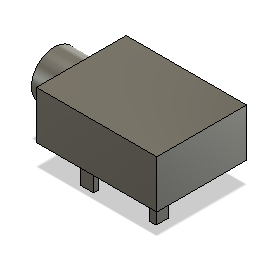
KTANE_game (Autodesk Fusion 360 archive; units mm, degrees)
design "3,5 mm female jack"
Autodesk Fusion 360 part; units mm, degrees
sketch "Sketch1" plane through (0, 0, 0) normal (0, 1, 0) x (1, 0, 0)
  line L0 (7.81, -5.825) -> (-7.81, -5.825)
  line L1 (-7.81, -5.825) -> (-7.81, 5.825)
  line L2 (-7.81, 5.825) -> (7.81, 5.825)
  line L3 (7.81, 5.825) -> (7.81, -5.825)
  line L4 (7.81, -5.825) -> (-7.81, 5.825) construction
  line L5 (-7.81, -5.825) -> (7.81, 5.825) construction
  dimension "d1" = 15.62
  dimension "d2" = 11.65
  constraint horizontal L0
  constraint perpendicular L0 L1
  constraint parallel L0 L2
  constraint parallel L1 L3
  constraint coincident L4 origin
  constraint coincident L5 origin
  measures "d1" distance of L1.end L2.end
  measures "d2" distance of L0.end L1.end
extrude "Extrude1" add sketch "Sketch1" along normal mid plane 6.2
sketch "Sketch2" plane through (-7.81, 0, 0) normal (-1, 0, 0) x (0, 0, 1)
  line L0 (5.825, -3.1) -> (5.825, 3.1)
  line L1 (5.825, 3.1) -> (-5.825, 3.1)
  line L2 (-5.825, 3.1) -> (-5.825, -3.1)
  line L3 (-5.825, -3.1) -> (5.825, -3.1)
  circle A0 centre (0, 0) radius 2.975
  circle A1 centre (0, 0) radius 1.8
  dimension "d5" = 5.95
  dimension "d6" = 3.6
  constraint coincident A0.centre A1.centre
  constraint concentric A0 A1
  measures "d5" diameter of A0
  measures "d6" diameter of A1
extrude "Extrude2" add sketch "Sketch2" along normal blind 3.5 contours A0
sketch "Sketch3" plane through (0, -3.1, 0) normal (0, -1, 0) x (1, 0, 0)
  line L0 (-7.81, -5.825) -> (7.81, -5.825)
  line L1 (7.81, -5.825) -> (7.81, 5.825)
  line L2 (7.81, 5.825) -> (-7.81, 5.825)
  line L3 (-7.81, 5.825) -> (-7.81, -5.825)
  line L4 (-1.1432, 4.3971) -> (-2.81, 4.3971)
  line L5 (-2.81, 4.3971) -> (-2.81, 5.075)
  line L6 (-2.81, 5.075) -> (-1.1432, 5.075)
  line L7 (-1.1432, 5.075) -> (-1.1432, 4.3971)
  line L8 (-1.1432, 4.3971) -> (-2.81, 5.075) construction
  line L9 (-2.81, 4.3971) -> (-1.1432, 5.075) construction
  line L10 (-5.2893, -1.2) -> (-6.2893, -1.2)
  line L11 (-6.2893, -1.2) -> (-6.2893, 1.2)
  line L12 (-6.2893, 1.2) -> (-5.2893, 1.2)
  line L13 (-5.2893, 1.2) -> (-5.2893, -1.2)
  line L14 (-5.2893, -1.2) -> (-6.2893, 1.2) construction
  line L15 (-6.2893, -1.2) -> (-5.2893, 1.2) construction
  line L16 (4.5993, -4.278) -> (2.9993, -4.278)
  line L17 (2.9993, -4.278) -> (2.9993, -3.678)
  line L18 (2.9993, -3.678) -> (4.5993, -3.678)
  line L19 (4.5993, -3.678) -> (4.5993, -4.278)
  line L20 (4.5993, -4.278) -> (2.9993, -3.678) construction
  line L21 (2.9993, -4.278) -> (4.5993, -3.678) construction
  line L22 (6.5448, 3.0401) -> (5.7448, 3.0401)
  line L23 (5.7448, 3.0401) -> (5.7448, 4.6401)
  line L24 (5.7448, 4.6401) -> (6.5448, 4.6401)
  line L25 (6.5448, 4.6401) -> (6.5448, 3.0401)
  line L26 (6.5448, 3.0401) -> (5.7448, 4.6401) construction
  line L27 (5.7448, 3.0401) -> (6.5448, 4.6401) construction
  point P0 (-1.9766, 4.736)
  point P1 (-5.7893, 0)
  point P2 (3.7993, -3.978)
  point P3 (6.1448, 3.8401)
  dimension "d9" = 1
  dimension "d10" = 2.4
  dimension "d15" = 5
  dimension "d16" = 0.75
  constraint horizontal L4
  constraint perpendicular L4 L5
  constraint parallel L4 L6
  constraint parallel L5 L7
  constraint coincident L8 P0
  constraint coincident L9 P0
  constraint horizontal L10
  constraint perpendicular L10 L11
  constraint parallel L10 L12
  constraint parallel L11 L13
  constraint coincident L14 P1
  constraint coincident L15 P1
  constraint horizontal L16
  constraint perpendicular L16 L17
  constraint parallel L16 L18
  constraint parallel L17 L19
  constraint coincident L20 P2
  constraint coincident L21 P2
  constraint horizontal L22
  constraint perpendicular L22 L23
  constraint parallel L22 L24
  constraint parallel L23 L25
  constraint coincident L26 P3
  constraint coincident L27 P3
  measures "d9" distance of L11.end L12.end
  measures "d10" distance of L10.end L11.end
  measures "d15" distance of L3 L5
  measures "d16" distance of L2 L6
extrude "Extrude3" add sketch "Sketch3" along normal blind 2.7 contours L4 L5 L6 L7 | L10 L11 L12 L13 | L16 L17 L18 L19 | L22 L23 L24 L25
extrude "Extrude4" cut 1 faces at (-7.81, 0.5565, 0.3541) along direction (1, 0, 0) blind 10.4
equation "d1 = 14.35 mm + 1.27 mm"
equation "d3 = ( 6.2 / 2 ) * 1 mm"
equation "d7 = 3.5 mm"
equation "d13 = -13.9 mm + d7"

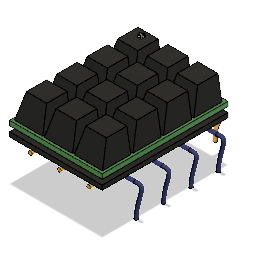
design "Keypad_component"
Autodesk Fusion 360 part; units mm, degrees
sketch "Sketch1" plane through (0, 0, 0) normal (0, 1, 0) x (1, 0, 0)
  line L0 (29.5, 40) -> (-29.5, 40)
  line L1 (-29.5, 40) -> (-29.5, -40)
  line L2 (-29.5, -40) -> (29.5, -40)
  line L3 (29.5, -40) -> (29.5, 40)
  line L4 (29.5, 40) -> (-29.5, -40) construction
  line L5 (-29.5, 40) -> (29.5, -40) construction
  line L6 (0, 40) -> (0, -40) construction
  line L7 (9, 19.6401) -> (-9, 19.6401)
  line L8 (-9, 19.6401) -> (-9, 37.6401)
  line L9 (-9, 37.6401) -> (9, 37.6401)
  line L10 (9, 37.6401) -> (9, 19.6401)
  line L11 (9, 19.6401) -> (-9, 37.6401) construction
  line L12 (-9, 19.6401) -> (9, 37.6401) construction
  point P0 (0, 28.6401)
  dimension "d6" = 59
  dimension "d7" = 80
  dimension "d11" = 18
  dimension "d12" = 18
  constraint horizontal L0
  constraint perpendicular L0 L1
  constraint parallel L0 L2
  constraint parallel L1 L3
  constraint coincident L4 origin
  constraint coincident L5 origin
  constraint midpoint L0 L6.start
  constraint midpoint L2 L6.end
  constraint horizontal L7
  constraint perpendicular L7 L8
  constraint parallel L7 L9
  constraint parallel L8 L10
  constraint coincident L11 P0
  constraint coincident L12 P0
  constraint coincident L6 P0
  measures "d6" distance of L1.end L2.end
  measures "d7" distance of L0.end L1.end
  measures "d11" distance of L8.end L9.end
  measures "d12" distance of L7.end L8.end
extrude "Extrude1" add sketch "Sketch1" against normal blind 3 contours L0 L1 L2 L3 | L7 L8 L9 L10 makes body 1
ref_plane "WorkPlane1" through (0, 14.5, 0) normal (0, -1, 0) x (0, 0, -1)
sketch "Sketch2" plane through (0, 14.5, 0) normal (0, -1, 0) x (-1, 0, 0)
  line L0 (9, 19.6401) -> (9, 37.6401)
  line L1 (-9, 37.6401) -> (9, 37.6401)
  line L2 (9, 19.6401) -> (-9, 19.6401)
  line L3 (-9, 37.6401) -> (-9, 19.6401)
  line L4 (0, 37.6401) -> (0, 19.6401) construction
  line L5 (-6.5, 37.6401) -> (6.5, 37.6401)
  line L6 (6.5, 37.6401) -> (6.5, 24.6401)
  line L7 (6.5, 24.6401) -> (-6.5, 24.6401)
  line L8 (-6.5, 24.6401) -> (-6.5, 37.6401)
  dimension "d14" = 13
  dimension "d15" = 13
  dimension "d16" = 6.5
  constraint midpoint L1 L4.start
  constraint midpoint L2 L4.end
  constraint horizontal L5
  constraint vertical L6
  constraint horizontal L7
  constraint vertical L8
  constraint coincident L1 L5.start
  measures "d14" distance of L5.start L5.end
  measures "d15" distance of L5.start L7.end
  measures "d16" distance of L4 L6
loft "Loft1" add profiles "Sketch1", "Sketch2" section 1 contours L7 L8 L9 L10 section 2 contours L1 L5 L6 L7 L8 separate body makes body 2
pattern_linear "R-Pattern1" count 4 spacing 19.3333 along (0, 0, 1) count 3 spacing 19 along (-1, 0, 0) both ways of bodies 2 makes body 3 at (-3, 0, -6.3067) makes body 4 at (-3, 0, 13.0266) makes body 5 at (-3, 0, 32.3599) makes body 6 at (22, 0, -25.6401) makes body 7 at (16, 0, -6.3067) makes body 8 at (16, 0, 13.0266) makes body 9 at (16, 0, 32.3599) makes body 10 at (-16, 0, -25.6401) makes body 11 at (-16, 0, -6.3067) makes body 12 at (-22, 0, 13.0266) makes body 13 at (-16, 0, 32.3599)
extrude "Extrude2" add sketch "Sketch1" against normal blind 3 from surface at -6.25 separate body contours L0 L1 L2 L3 | L7 L8 L9 L10 makes body 14
sketch "Sketch3" plane through (0, 14.5, 0) normal (0, 1, 0) x (-1, 0, 0)
  line L0 (12.5, -37.6401) -> (25.5, -37.6401)
  line L1 (25.5, -37.6401) -> (25.5, -24.6401)
  line L2 (25.5, -24.6401) -> (12.5, -24.6401)
  line L3 (12.5, -24.6401) -> (12.5, -37.6401)
  line L4 (25.5, -24.6401) -> (12.5, -24.6401) construction
  line L5 (12.5, -24.6401) -> (12.5, -37.6401) construction
  line L6 (12.5, -37.6401) -> (25.5, -37.6401) construction
  line L7 (25.5, -37.6401) -> (25.5, -24.6401) construction
  dimension "d24" = 8
  text T0 "*" font "Arial" height 8 align centre middle in box 13 x 13 at (25.5, -24.6401) x (-1, 0) y (0, -1) spacing 1 kerned
  constraint coincident L0.start
  constraint coincident L1.end
extrude "Extrude3" add sketch "Sketch3" along normal blind 1 text T0 bodies 10
sketch "Sketch4" plane through (0, 0, -40) normal (0, 0, -1) x (-1, 0, 0)
  line L0 (29.5, -6.25) -> (-29.5, -6.25)
  line L1 (-29.5, -6.25) -> (-29.5, -9.25)
  line L2 (-29.5, -9.25) -> (29.5, -9.25)
  line L3 (29.5, -9.25) -> (29.5, -6.25)
  circle A0 centre (-2.2, -11.5) radius 1.25
  line L4 (0, 0) -> (0, -6.25) construction
  dimension "d29" = 2.5
  dimension "d30" = 2.25
  dimension "d33" = 18.5
  dimension "d34" = 0
  dimension "d35" = 2.2
  constraint coincident L4.start origin
  constraint midpoint L0 L4.end
  measures "d29" diameter of A0
  measures "d30" distance of L2 A0.centre
  measures "d35" distance of A0.centre L4
extrude "Extrude4" add sketch "Sketch4" against normal up to surface (80 mm away) separate body contours A0 makes body 15
sketch "Sketch5" plane through (0, 0, 0) normal (1, 0, 0) x (0, 0, -1)
  line L0 (40, -12.75) -> (40, -10.25)
  line L1 (45, -14) -> (43, -17) construction
  spline S0 degree 5 poles (40, -11.5) (40.28, -11.496) (40.8403, -11.5188) (41.6814, -11.6456) (42.7775, -11.9864) (43.9626, -12.6229) (44.7996, -13.3774) (45.1587, -14.1634) (45.0061, -14.9254) (44.4446, -15.6571) (43.6435, -16.3858) (42.7906, -17.1632) (42.0322, -18.0537) (41.4348, -19.1264) (41.0134, -20.4507) (40.7479, -22.0918) (40.6312, -23.7028) (40.5817, -25.0966) (40.5632, -26.1104) (40.5576, -26.6385) knots 0 0 0 0 0 0 0.066667 0.133333 0.2 0.266667 0.333333 0.4 0.466667 0.533333 0.6 0.666667 0.733333 0.8 0.866667 0.933333 1 1 1 1 1 1 construction
  line L2 (37.2978, -11.5388) -> (42.7022, -11.4612)
  line L3 (40.5988, -22.7617) -> (40.5163, -30.5153)
  constraint midpoint L0 S0.start
  constraint midpoint S0.start L2
  constraint midpoint S0.end L3
sweep "Sweep1" add 1 faces at (1.8946, -10.971, -40) path "Sketch5" along S0 on bodies 15 bodies 15
pattern_linear "R-Pattern2" count 3 spacing 18.5 along (-1, 0, 0) both ways of bodies 15 makes body 16 at (19.4516, -11.5623, 13.3333) makes body 17 at (-17.5484, -11.5623, 13.3333)
sketch "Sketch6" plane through (29.5, 0, 0) normal (1, 0, 0) x (0, 0, -1)
  line L0 (40, -6.25) -> (-40, -6.25)
  line L1 (-40, -6.25) -> (-40, -9.25)
  line L2 (-40, -9.25) -> (40, -9.25)
  line L3 (40, -9.25) -> (40, -6.25)
  circle A0 centre (33.25, -14.9) radius 1.25
  dimension "d48" = 2.5
  dimension "d49" = 5.65
  dimension "d50" = 6.75
  measures "d48" diameter of A0
  measures "d49" distance of L2 A0.centre
  measures "d50" distance of L3 A0.centre
extrude "Extrude5" add sketch "Sketch6" against normal up to surface (59 mm away) separate body contours A0 makes body 18
sketch "Sketch7" plane through (0, 0, 0) normal (0, 0, 1) x (1, 0, 0)
  line L0 (29.5, -16.15) -> (29.5, -13.65)
  spline S0 degree 5 poles (29.5, -14.9) (29.6524, -14.8992) (29.9786, -14.8935) (30.532, -14.8721) (31.3601, -14.8468) (32.3535, -14.9634) (33.0985, -15.3824) (33.4753, -16.1914) (33.486, -17.3855) (33.1998, -18.909) (32.7243, -20.6767) (32.1686, -22.6017) (31.6106, -24.6193) (31.1012, -26.6848) (30.6714, -28.7689) (30.3373, -30.8544) (30.1514, -32.5174) (30.058, -33.7603) (30.0159, -34.5871) (30, -35) knots 0 0 0 0 0 0 0.066667 0.133333 0.2 0.266667 0.333333 0.4 0.466667 0.533333 0.6 0.666667 0.733333 0.8 0.866667 0.933333 1 1 1 1 1 1
  line L1 (28.0397, -14.9073) -> (30.9603, -14.8927)
  point P0 (32.7337, -15.2452)
  point P1 (32.6845, -20.7869)
  constraint midpoint L0 S0.start
  constraint midpoint S0.start L1
sweep "Sweep2" add 1 faces at (29.5, -15.7757, -33.1573) path "Sketch7" along S0 on bodies 18 bodies 18
pattern_linear "R-Pattern3" count 4 spacing 17.4 along (0, 0, 1) of bodies 18 makes body 19 at (-9.8333, -14.9623, -17.0984) makes body 20 at (-9.8333, -14.9623, 0.3016) makes body 21 at (-9.8333, -14.9623, 17.7016)
equation "keypad_width = 59 mm"
equation "keypad_length = 80 mm"
equation "keycap_width = 18 mm"
equation "keycap_lenght = 18 mm"
equation "keycap_height = 17.5 mm"
equation "d6 = keypad_width"
equation "d7 = keypad_length"
equation "bottom_keypad_thickness = 3 mm"
equation "d9 = -bottom_keypad_thickness"
equation "d11 = keycap_lenght"
equation "d12 = keycap_width"
equation "d13 = -keycap_height"
equation "d16 = d14 / 2"
equation "d21 = -3.25 mm - bottom_keypad_thickness"
equation "d22 = -bottom_keypad_thickness"
equation "wire_width = 2.5 mm"
equation "d29 = wire_width"
equation "d30 = d29 / 2 + 1 mm"
equation "d48 = wire_width"
equation "d49 = d48 / 2 + 4.4 mm"
equation "d50 = d48 / 2 + 5.5 mm"
named bodies: "Green_bottom", "Black_bottom"

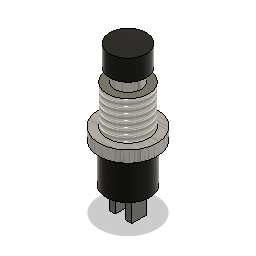
design "Small push-button"
Autodesk Fusion 360 part; units mm, degrees
sketch "Sketch1" plane through (0, 0, 0) normal (0, 1, 0) x (1, 0, 0)
  circle A0 centre (0, 0) radius 4.8
  dimension "d6" = 9.6
  constraint coincident A0.centre origin
  measures "d6" diameter of A0
extrude "Extrude1" add sketch "Sketch1" along normal mid plane 1.9
sketch "Sketch2" plane through (0, 0.95, 0) normal (0, 1, 0) x (-1, 0, 0)
  circle A0 centre (0, 0) radius 4.8
  circle A1 centre (0, 0) radius 3.385
  dimension "d9" = 6.77
  constraint coincident A0.centre A1.centre
  measures "d9" diameter of A1
extrude "Extrude2" add sketch "Sketch2" along normal blind 6.4 contours A1
sketch "Sketch3" plane through (0, 7.35, 0) normal (0, 1, 0) x (-1, 0, 0)
  circle A0 centre (0, 0) radius 3.385
  circle A1 centre (0, 0) radius 2.165
  dimension "d12" = 4.33
  constraint concentric A0 A1
  measures "d12" diameter of A1
extrude "Extrude3" add sketch "Sketch3" along normal blind 2.09 contours A1
sketch "Sketch4" plane through (0, 9.44, 0) normal (0, 1, 0) x (-1, 0, 0)
  circle A0 centre (0, 0) radius 2.165
  circle A1 centre (0, 0) radius 3.035
  dimension "d15" = 6.07
  constraint concentric A0 A1
  measures "d15" diameter of A1
extrude "Extrude4" add sketch "Sketch4" along normal blind 3.44 contours A0 | A1
sketch "Sketch5" plane through (0, -0.95, 0) normal (0, -1, 0) x (1, 0, 0)
  circle A0 centre (0, 0) radius 4.8
  circle A1 centre (0, 0) radius 3.615
  dimension "d18" = 7.23
  constraint concentric A0 A1
  measures "d18" diameter of A1
extrude "Extrude5" add sketch "Sketch5" along normal blind 6.5 contours A1
sketch "Sketch6" plane through (0, -7.45, 0) normal (0, -1, 0) x (1, 0, 0)
  circle A0 centre (0, 0) radius 3.615
  line L0 (-1.865, 1.25) -> (-0.865, 1.25)
  line L1 (-0.865, 1.25) -> (-0.865, -1.25)
  line L2 (-0.865, -1.25) -> (-1.865, -1.25)
  line L3 (-1.865, -1.25) -> (-1.865, 1.25)
  line L4 (-3.615, 0) -> (3.615, 0) construction
  line L5 (0, 1.75) -> (0, 22.5)
  dimension "d21" = 2.5
  dimension "d22" = 1.25
  dimension "d23" = 1.75
  dimension "d24" = 1
  constraint horizontal L0
  constraint vertical L1
  constraint horizontal L2
  constraint vertical L3
  constraint coincident A0 L4.start
  constraint coincident A0 L4.end
  constraint perpendicular L4 L5
  constraint coincident A0.centre L4
  measures "d21" distance of L0.end L1.end
  measures "d22" distance of L2 L4
  measures "d23" distance of L3 L4.start
  measures "d24" distance of L0.start L0.end
extrude "Extrude6" add sketch "Sketch6" along normal blind 4 contours L0 L1 L2 L3
mirror "Mirror1" about plane through (0, 0, 0) normal (1, 0, 0) of "Extrude6"
thread "Thread1" "ISO Metric profile 7.0 M7x1 6g" major diameter 6.884 minor diameter 5.744 pitch 1 angle 60 resizes the face on face at (-3.3808, 5.2167, -0.1687)
equation "button_ring = 9.6 mm"
equation "button_threaded_cylinder_diameter = 6.77 mm"
equation "button_black_cylinder_diameter = 7.23 mm"
equation "button_cylinder_between_button_and_top_diameter = 4.33 mm"
equation "button_top_diameter = 6.07 mm"
equation "d6 = button_ring"
equation "d7 = 1.9 mm / 2"
equation "d9 = button_threaded_cylinder_diameter"
equation "d12 = button_cylinder_between_button_and_top_diameter"
equation "d15 = button_top_diameter"
equation "d18 = button_black_cylinder_diameter"
equation "d22 = d21 / 2"
